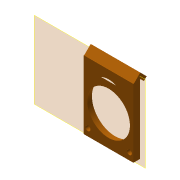
# Autodesk Inventor part: 30_Cube_Insert_Filter_Revolver_Filter_lid_linearmotor
Saved by Autodesk Inventor 2022 (Build 260153000, 153)
## iProperties
Created: 2021-12-21
Part Number: 30_Cube_Insert_Filter_Revolver_Filter_lid_linearmotor
Material: Generisch
Document SubType Name: Modeling
Designer: diederichbenedict
Density: 1 g/cm^3
Appearance: Orange
Author: diederichbenedict
Autodesk Inventor part; units mm, degrees
ref_plane "YZ Plane" through (0, 0, 0) normal (1, 0, 0) x (0, 1, 0)
ref_plane "XZ Plane" through (0, 0, 0) normal (0, 1, 0) x (-1, 0, 0)
ref_plane "XY Plane" through (0, 0, 0) normal (0, 0, 1) x (1, 0, 0)
ref_plane "Arbeitsebene1" through (0, 0, 0) normal (0, 0, 1) x (1, 0, 0)
sketch "Skizze1" plane through (0, 0, 0) normal (0, 0, 1) x (1, 0, 0)
  line L0 (-17.0991, 11.5492) -> (-20.941, 11.5492) projected
  ellipse E0 centre (-28, 1.5322) end of major axis (-28, -12.6099) minor radius 10 (-35.059, 11.5492) -> (-20.941, 11.5492) ccw projected
  line L1 (-35.059, 11.5492) -> (-38.9009, 11.5492) projected
  ellipse E1 centre (-28, 1.5322) end of major axis (-28, 19.917) minor radius 13 (-17.0991, 11.5492) -> (-38.9009, 11.5492) ccw projected
  circle A0 centre (-39.5, -12.9132) radius 1.4 projected
  circle A1 centre (-16.5, -12.9132) radius 1.4 projected
  line L2 (14, -17.9132) -> (-42, -17.9132) projected
  line L3 (14, 20.9777) -> (14, -17.9132) projected
  line L4 (-42, 20.9777) -> (14, 20.9777) projected
  line L5 (-42, -17.9132) -> (-42, 20.9777) projected
  line L6 (10.9009, 11.5492) -> (7.059, 11.5492) projected
  ellipse E2 centre (0, 1.1319) end of major axis (0, -13.1363) minor radius 10.3303 (-7.059, 11.5492) -> (7.059, 11.5492) ccw
  line L7 (-7.059, 11.5492) -> (-10.9009, 11.5492) projected
  ellipse E3 centre (0, 1.058) end of major axis (-0.0732, 16.1871) minor radius 15.1293 (10.9009, 11.5492) -> (-10.9009, 11.5492) ccw
  circle A2 centre (-11.5, -12.9132) radius 1.4 projected
  circle A3 centre (11.5, -12.9132) radius 1.4 projected
  line L8 (13.75, 22.4777) -> (-13.75, 22.4777)
  line L9 (-13.75, 22.4777) -> (-13.75, -16.9132)
  line L10 (-13.75, -16.9132) -> (13.75, -16.9132)
  line L11 (13.75, -16.9132) -> (13.75, 22.4777)
  line L12 (13.75, 22.4777) -> (-13.75, -16.9132) construction
  line L13 (-13.75, 22.4777) -> (13.75, -16.9132) construction
  circle A4 centre (0, 0) radius 12.85
  point P0 (0, 0)
  point P1 (0, 2.7822)
  point P2 (13.75, 20.9777)
  point P3 (-13.75, 20.9777)
  dimension "d0" = 27.5
  dimension "d1" = 4
  dimension "d2" = 1.5
  dimension "d3" = 25.7
  constraints: 12 end point, 2 midpoint, 2 parallel, 1 centre point, 1 coincident, 1 horizontal, 1 perpendicular, 10 other
  measures "d0" distance of L10.end L9.end
  measures "d1" distance from line of A2.centre L10
  measures "d2" distance between parallel lines of L8 L4
  measures "d3" diameter of A4
extrude "Extrusion1" add sketch "Skizze1" along normal blind 3.3 contours L11 L10 L9 L4 | L6 E2 A4 L7 E3 | E2 A4 picked at (0.149, -12.9119)
sketch "Skizze2" plane through (13.75, -16.9132, 0) normal (1, 0, 0) x (0, 0, -1)
  line L0 (0, 0) -> (0, 37.8909) projected
  line L1 (0, 37.8909) -> (-3.3, 37.8909) projected
  line L2 (-3.3, 0) -> (-3.3, 37.8909) projected
  line L3 (0, 0) -> (-3.3, 0) projected
  circle A0 centre (6.0056, 17.0971) radius 1.635 projected
  line L4 (0, -1) -> (5.3033, -6.3033) projected
  line L5 (5.3033, -6.3033) -> (12.9197, 1.3131) projected
  arc A1 (14.8458, 3.2392) -> (12.9197, 1.3131) centre (13.3595, 2.7994) ccw projected
  line L6 (14.8458, 3.2392) -> (15.8697, 4.2631) projected
  line L7 (15.8697, 4.2631) -> (12.6948, 7.438) projected
  arc A2 (15.6647, 10.4079) -> (12.6948, 7.438) centre (14.1797, 8.923) ccw projected
  line L8 (15.6647, 10.4079) -> (18.8396, 7.233) projected
  line L9 (18.8396, 7.233) -> (19.8635, 8.2569) projected
  arc A3 (21.7896, 10.183) -> (19.8635, 8.2569) centre (20.3033, 9.7432) ccw projected
  line L10 (21.7896, 10.183) -> (24.9843, 13.3777) projected
  line L11 (24.9843, 13.3777) -> (0.2355, 38.1264) projected
  line L12 (0.2355, 38.1264) -> (0, 37.8909) projected
  line L13 (0, 37.8909) -> (0, -1) projected
  line L14 (-3.3, 0) -> (-3.3, 37.8909) projected
  line L15 (-3.3, 37.8909) -> (0.2355, 41.4264)
  line L16 (0.2355, 41.4264) -> (3.7711, 37.8909)
  line L17 (3.7711, 37.8909) -> (2.1211, 36.2409)
  line L18 (0, 0) -> (0, 37.8909) projected
  line L19 (0, 37.8909) -> (0.3416, 38.2325)
  line L20 (0.3416, 38.2325) -> (2.2271, 36.3469)
  point P0 (0, 16.9132)
  point P1 (0.2355, 38.1264)
  dimension "d6" = 5
  dimension "d7" = 5
  dimension "d8" = 0.15
  constraints: 10 end point, 4 perpendicular, 2 point on line
  measures "d6" distance of L1.end L15.end
  measures "d7" distance of L15.end L16.end
  measures "d8" distance between parallel lines of L11 L20
extrude "Extrusion2" add sketch "Skizze2" against normal up to surface (27.5 mm away) contours L1 L15 L16 L17 L20 L19 L12
sketch "Skizze3" plane through (0, 0, 3.3) normal (0, 0, 1) x (1, 0, 0)
  line L0 (13.75, -16.9132) -> (13.75, 20.9777) projected
  line L1 (13.75, 20.9777) -> (-13.75, 20.9777) projected
  line L2 (-13.75, 20.9777) -> (-13.75, -16.9132) projected
  line L3 (-13.75, -16.9132) -> (13.75, -16.9132) projected
  circle A0 centre (0, 0) radius 12.85 projected
  circle A1 centre (11.5, -12.9132) radius 1.4 projected
  circle A2 centre (-11.5, -12.9132) radius 1.4 projected
  circle A3 centre (0, 0) radius 11.85
  point P0 (0, 0)
  dimension "d11" = 1
  constraints: 1 centre point
  measures "d11" radial gap between concentric circles of A0 A3
extrude "Extrusion3" add sketch "Skizze3" along normal blind 0.3 contours L3 L2 L1 L0 | A0
sketch "Skizze4" plane through (-13.75, 19.4337, -2.2271) normal (0, -0.7071068, 0.7071068) x (1, 0, 0)
  circle A0 centre (13.75, -11.0835) radius 13 projected
  point P0 (13.75, -12.1669)
extrude "Extrusion4" cut sketch "Skizze4" along normal blind 7
sketch "Skizze5" plane through (13.75, 24.5132, -0.2355) normal (0, 0.7071068, -0.7071068) x (-1, 0, 0)
  circle A0 centre (13.75, -16.0835) radius 13 projected
  point P0 (13.75, -17.1669)
extrude "Extrusion5" cut sketch "Skizze5" against normal up to surface (2.1835 mm away)
